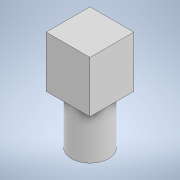
# Autodesk Inventor part: Motor_Key_Bearing_2_2
Saved by Autodesk Inventor 2022 (Build 260153000, 153)
## iProperties
Created: 2023-02-21
Part Number: Motor_Key_Bearing_2_2
Material: Generic
Document SubType Name: Modeling
Designer: zarek
Density: 1 g/cm^3
Appearance: Default
Author: zarek
Autodesk Inventor part; units mm, degrees
ref_plane "YZ Plane" through (0, 0, 0) normal (1, 0, 0) x (0, 1, 0)
ref_plane "XZ Plane" through (0, 0, 0) normal (0, 1, 0) x (-1, 0, 0)
ref_plane "XY Plane" through (0, 0, 0) normal (0, 0, 1) x (1, 0, 0)
sketch "Sketch1" plane through (0, 0, 0) normal (0, 1, 0) x (-1, 0, 0)
  line L0 (14.5, -14.5) -> (-14.5, -14.5)
  line L1 (-14.5, -14.5) -> (-14.5, 14.5)
  line L2 (-14.5, 14.5) -> (14.5, 14.5)
  line L3 (14.5, 14.5) -> (14.5, -14.5)
  circle A0 centre (0, 0) radius 4
  dimension "d11" = 29
  dimension "d14" = 29
  dimension "d31" = 8
  constraints: 8 end point, 2 parallel, 1 centre point, 1 horizontal, 1 perpendicular
  measures "d11" distance between parallel lines of L1 L3
  measures "d14" distance between parallel lines of L2 L0
  measures "d31" diameter of A0
extrude "Extrusion1" add sketch "Sketch1" along normal blind 10.5 contours A0
sketch "Sketch2" plane through (0, 10.5, 0) normal (0, 1, 0) x (1, 0, 0)
  line L0 (-4.7, 4.7) -> (4.7, 4.7)
  line L1 (4.7, 4.7) -> (4.7, -4.7)
  line L2 (4.7, -4.7) -> (-4.7, -4.7)
  line L3 (-4.7, -4.7) -> (-4.7, 4.7)
  line L4 (14.5, 14.5) -> (-14.5, 14.5) projected
  line L5 (14.5, -14.5) -> (14.5, 14.5) projected
  line L6 (-14.5, -14.5) -> (14.5, -14.5) projected
  line L7 (-14.5, 14.5) -> (-14.5, -14.5) projected
  point P0 (0, 0)
  dimension "d15" = 9.8
  dimension "d16" = 9.8
  dimension "d17" = 9.8
  dimension "d18" = 9.8
  dimension "d32" = 9.4
  dimension "d50" = 29
  constraints: 8 end point, 2 parallel, 1 horizontal, 1 perpendicular
  measures "d15" distance between parallel lines of L0 L4
  measures "d16" distance between parallel lines of L5 L1
  measures "d17" distance between parallel lines of L6 L2
  measures "d18" distance between parallel lines of L7 L3
  measures "d32" distance between parallel lines of L1 L3
  measures "d50" distance between parallel lines of L6 L4
extrude "Extrusion2" add sketch "Sketch2" along normal blind 11 contours L0 L1 L2 L3
sketch "Sketch3" plane through (0, 0, 0) normal (0, -1, 0) x (1, 0, 0)
  line L0 (-0.0005, -0.0003) -> (-0.0005, -1.7003)
  line L1 (-0.0005, -1.7003) -> (2.6995, -1.7003)
  line L2 (2.6995, -1.7003) -> (2.6995, 1.6997)
  line L3 (2.6995, 1.6997) -> (-2.7005, 1.6997)
  line L4 (-2.7005, 1.6997) -> (-2.7005, -1.7003)
  line L5 (-2.7005, -1.7003) -> (-0.0005, -1.7003)
  dimension "d42" = 1.7
  dimension "d43" = 2.7
  dimension "d44" = 3.4
  dimension "d45" = 5.4
  constraints: 12 end point, 5 perpendicular, 1 point on line, 1 vertical
  measures "d42" distance of L0.start L0.end
  measures "d43" distance of L0.end L1.end
  measures "d44" distance of L1.end L2.end
  measures "d45" distance of L2.end L3.end
extrude "Extrusion3" cut sketch "Sketch3" against normal blind 8.2
sketch "Sketch5" plane through (0, 0, 0) normal (0, -1, 0) x (1, 0, 0)
  circle A0 centre (0, 0) radius 2.7
  dimension "d35" = 5.4
  constraints: 1 centre point, 1 coincident
  measures "d35" diameter of A0
extrude "Extrusion4" cut sketch "Sketch5" against normal blind 2.2
fillet "Fillet1" radius 0.635 4 edges at (2.6995, 4.1, 1.6997) (2.6995, 4.1, -1.7003) (-2.7005, 4.1, -1.7003) (-2.7005, 4.1, 1.6997)
equation "\"d14\" = d11"
equation "\"d16\" = d15"
equation "\"d17\" = d15"
equation "\"d18\" = d15"
equation "\"d42\" = 0.5 * d44"
body "Solid1"
